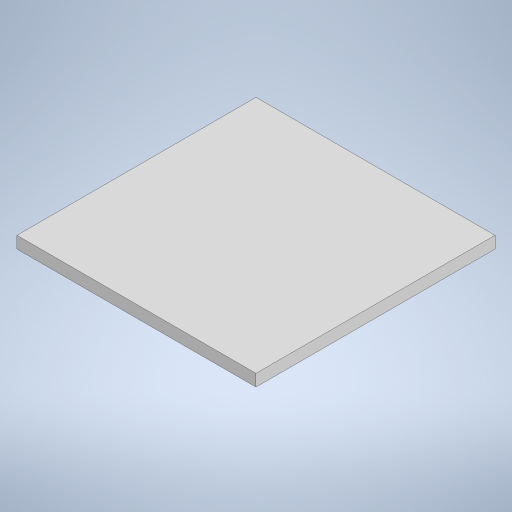
# Autodesk Inventor part: Front_base
Saved by Autodesk Inventor 2024 (Build 280153000, 153)
## iProperties
Created: 2023-12-18
Part Number: Front_base
Material: Generic
Document SubType Name: Modeling
Designer: Mechatronics Lab 1
Density: 1 g/cm^3
Appearance: Default
Author: Mechatronics Lab 1
Autodesk Inventor part; units mm, degrees
ref_plane "YZ Plane" through (0, 0, 0) normal (1, 0, 0) x (0, 1, 0)
ref_plane "XZ Plane" through (0, 0, 0) normal (0, 1, 0) x (-1, 0, 0)
ref_plane "XY Plane" through (0, 0, 0) normal (0, 0, 1) x (1, 0, 0)
sketch "Sketch46" plane through (0, 0, 0) normal (0, 1, 0) x (-1, 0, 0)
  circle A0 centre (0, 0) radius 1.5
  dimension "d158" = 3
  constraints: 1 centre point, 1 coincident
  measures "d158" diameter of A0
extrude "Extrusion35" add sketch "Sketch46" along normal blind 3
sketch "Sketch47" plane through (0, 3, 0) normal (0, 1, 0) x (1, 0, 0)
  line L0 (-20, 20) -> (20, 20)
  line L1 (20, 20) -> (20, -20)
  line L2 (20, -20) -> (-20, -20)
  line L3 (-20, -20) -> (-20, 20)
  line L4 (-20, 20) -> (20, -20) construction
  line L5 (20, 20) -> (-20, -20) construction
  point P0 (0, 0)
  dimension "d161" = 40
  dimension "d162" = 40
  constraints: 12 end point, 2 midpoint, 2 parallel, 1 horizontal, 1 perpendicular
  measures "d161" distance of L1.end L2.end
  measures "d162" distance of L0.end L1.end
extrude "Extrusion36" add sketch "Sketch47" along normal blind 2
sketch "Sketch48" plane through (0, 0, 0) normal (0, -1, 0) x (1, 0, 0)
  circle A0 centre (0, 0) radius 1.875
  dimension "d165" = 3.75
  constraints: 1 centre point, 1 coincident
  measures "d165" diameter of A0
extrude "Extrusion37" add sketch "Sketch48" along normal blind 1
body "Solid4"
